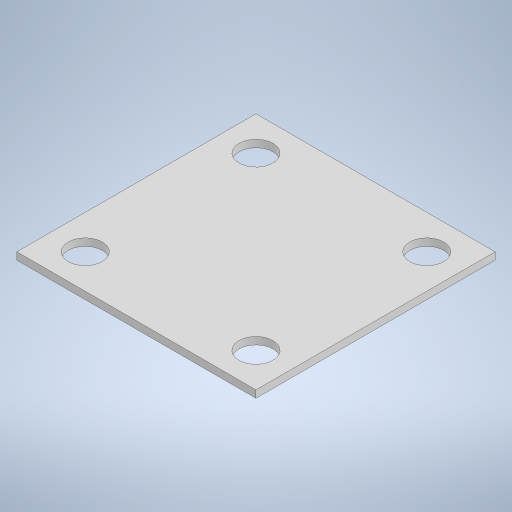
# Autodesk Inventor part: Plate1
Saved by Autodesk Inventor 2024.1 (Build 281209000, 209)
## iProperties
Created: 2023-12-23
Part Number: Plate1
Material: Generic
Document SubType Name: Modeling
Designer: ryanm
Density: 1 g/cm^3
Appearance: Default
Author: ryanm
Autodesk Inventor part; units mm, degrees
ref_plane "YZ Plane" through (0, 0, 0) normal (1, 0, 0) x (0, 1, 0)
ref_plane "XZ Plane" through (0, 0, 0) normal (0, 1, 0) x (-1, 0, 0)
ref_plane "XY Plane" through (0, 0, 0) normal (0, 0, 1) x (1, 0, 0)
sketch "Sketch1" plane through (0, 0, 0) normal (0, 1, 0) x (-1, 0, 0)
  line L0 (49, -49) -> (-49, -49)
  line L1 (-49, -49) -> (-49, 49)
  line L2 (-49, 49) -> (49, 49)
  line L3 (49, 49) -> (49, -49)
  circle A0 centre (35, -35) radius 7
  circle A1 centre (-35, -35) radius 7
  circle A2 centre (-35, 35) radius 7
  circle A3 centre (35, 35) radius 7
  point P0 (0, 0)
  point P1 (0, -49)
  point P2 (49, 0)
  dimension "d0" = 98
  dimension "d1" = 98
  dimension "d2" = 14
  dimension "d3" = 14
  dimension "d4" = 14
  dimension "d5" = 14
  dimension "d6" = 14
  dimension "d7" = 14
  dimension "d8" = 14
  dimension "d9" = 14
  constraints: 8 end point, 4 centre point, 3 horizontal alignment, 3 vertical alignment, 2 midpoint, 2 parallel, 1 horizontal, 1 perpendicular
  measures "d0" distance of L0.start L0.end
  measures "d1" distance of L2.end L0.start
  measures "d2" diameter of A0
  measures "d3" diameter of A1
  measures "d4" diameter of A3
  measures "d5" diameter of A2
  measures "d6" distance from line of L3 A0.centre
  measures "d7" distance from line of L0 A0.centre
  measures "d8" distance from line of L1 A2.centre
  measures "d9" distance from line of L2 A2.centre
extrude "Extrusion1" add sketch "Sketch1" along normal blind 3
equation "\"d3\" = d2"
equation "\"d4\" = d2"
equation "\"d5\" = d2"
equation "\"d8\" = d6"
equation "\"d9\" = d7"
body "Solid1"
